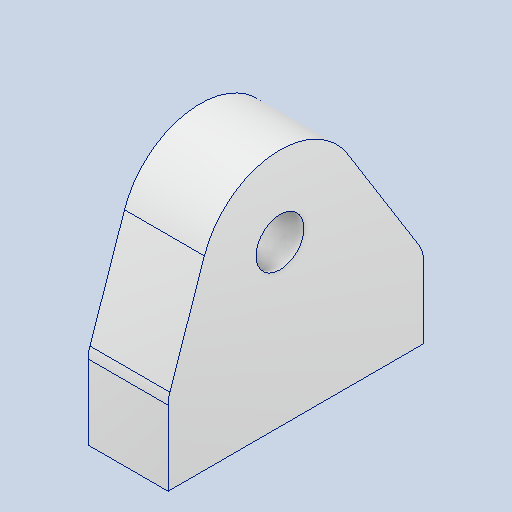
# Autodesk Inventor part: belt_liner_v5_Plate_10
Saved by Autodesk Inventor 2025.2 (Build 292293000, 293)
## iProperties
Created: 2025-02-23
Part Number: belt_liner_v5_Plate_10
Material: アルミニウム 6061
Document SubType Name: Modeling
Designer: haruy
Density: 2.7 g/cm^3
Appearance: アルミニウム - フラット
Author: haruy
Autodesk Inventor part; units mm, degrees
ref_plane "YZ Plane" through (0, 0, 0) normal (1, 0, 0) x (0, 1, 0)
ref_plane "XZ Plane" through (0, 0, 0) normal (0, 1, 0) x (-1, 0, 0)
ref_plane "XY Plane" through (0, 0, 0) normal (0, 0, 1) x (1, 0, 0)
sketch "スケッチ1" plane through (0, 0, 0) normal (1, 0, 0) x (0, 1, 0)
  circle A0 centre (0, 0) radius 5
  line L0 (5, 24) -> (-10, 24)
  line L1 (-10, 24) -> (-10, 9)
  line L2 (-10, 9) -> (5, 9)
  line L3 (5, 9) -> (5, 24)
  line L4 (-10, 9) -> (-15, 9)
  line L5 (-15, 9) -> (-15, -9)
  line L6 (-15, -9) -> (-10, -9)
  line L7 (-10, -9) -> (-10, 9)
  line L8 (-10, 9) -> (1.724, 4.6934)
  line L9 (1.724, -4.6934) -> (-10, -9)
  circle A1 centre (0, 0) radius 1.5
  line L10 (-10, 9) -> (-5, 9)
  line L11 (-5, 9) -> (-5, -9)
  line L12 (-5, -9) -> (-10, -9)
  line L13 (-10, -9) -> (-10, 9)
  line L14 (-5, 9) -> (2.6415, 4.2453)
  line L15 (-5, -9) -> (2.6415, -4.2453)
  line L16 (-5, 7) -> (-10, 7)
  line L17 (-5, 7) -> (1.6216, 4.7297)
  dimension "d0" = 10
  dimension "d1" = 15
  dimension "d2" = 15
  dimension "d3" = 5
  dimension "d5" = 18
  dimension "d6" = 3
  dimension "d7" = 10
  dimension "d8" = 9
  dimension "d11" = 5
  dimension "d12" = 18
  dimension "d29" = 2
  constraints: 36 end point, 7 parallel, 5 point on circle, 5 tangent, 3 horizontal, 3 perpendicular, 2 centre point, 2 coincident, 2 point on line
  measures "d0" diameter of A0
  measures "d1" distance of L2.end L1.end
  measures "d2" distance of L1.end L0.end
  measures "d3" distance of L6.end L5.end
  measures "d5" distance between parallel lines of L2 L6
  measures "d6" diameter of A1
  measures "d7" distance from line of L7 point (0, 0)
  measures "d8" distance from line of L2 point (0, 0)
  measures "d11" distance of L11.end L12.end
  measures "d12" distance between parallel lines of L2 L12
  measures "d29" distance from line of L10 L16.start
extrude "押し出し2" add sketch "スケッチ1" along normal blind 5 contours A0 | A0 L8 L11 L14 | L15 L11 L9 A0 | L11 L8 L2 | L9 L11 A0 | L12 L9 L11 | L17 L11 L8 | A0 L11 L17 | L8 L11 L16 L7 | L11 L9 L7 L16
fillet "フィレット1" radius 2 2 edges at (2.5, -5, -9) (2.5, -5, 9)
sketch "スケッチ2" plane through (0, -10, -9) normal (0, -1, 0) x (1, 0, 0)
  circle A0 centre (2.5, 3.5) radius 1.25
  line L0 (0, 0) -> (5, 0) projected
  line L1 (0, 18) -> (0, 0) projected
  circle A1 centre (2.5, 10.5) radius 1.25
  point P0 (0, 9)
  dimension "d16" = 2.5
  dimension "d17" = 3.5
  dimension "d18" = 2.5
  dimension "d19" = 2.5
  dimension "d20" = 2.5
  dimension "d21" = 7
  constraints: 2 centre point
  measures "d16" diameter of A0
  measures "d17" distance from line of A0.centre L0
  measures "d18" distance from line of A0.centre L1
  measures "d19" diameter of A1
  measures "d20" distance from line of A1.centre L1
  measures "d21" distance of A0.centre A1.centre
hole "穴1" at (2.5, -10, 1.5) at (2.5, -10, -5.5) direction (0, 1, 0) diameter 2.5 depth 5 tip angle 118
extrude "押し出し3" cut sketch "スケッチ1" along normal blind 10 contours A0 L8 L11 L14 | L11 L8 L2 | L17 L11 L8 | L8 L11 L16 L7
fillet "フィレット2" radius 2 1 edges at (2.5, -5, 7)
equation "\"d12\" = d5"
equation "\"d18\" = d16"
equation "\"d20\" = d18"
